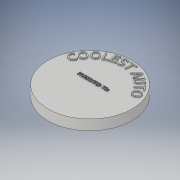
# Autodesk Inventor part: COOLEST AUTO
Saved by Autodesk Inventor 2018.2 (Build 222227000, 227)
## iProperties
Created: 2018-03-08
Part Number: COOLEST AUTO
Material: Generic
Document SubType Name: Modeling
Designer: battin.michael
Density: 1 g/cm^3
Appearance: Default
Author: battin.michael
Autodesk Inventor part; units mm, degrees
ref_plane "YZ Plane" through (0, 0, 0) normal (1, 0, 0) x (0, 1, 0)
ref_plane "XZ Plane" through (0, 0, 0) normal (0, 1, 0) x (-1, 0, 0)
ref_plane "XY Plane" through (0, 0, 0) normal (0, 0, 1) x (1, 0, 0)
sketch "Sketch1" plane through (0, 0, 0) normal (0, 1, 0) x (-1, 0, 0)
  circle A0 centre (0, 0) radius 104.775
  dimension "d0" = 209.55
  constraints: 1 centre point, 1 coincident
  measures "d0" diameter of A0
extrude "Extrusion1" add sketch "Sketch1" along normal blind 25.4
sketch "Sketch2" plane through (0, 25.4, 0) normal (0, 1, 0) x (1, 0, 0)
  circle A0 centre (0, 0) radius 104.775
  spline S0 degree 2 poles (-70.4833, 32.8422) (-71.2808, 31.0342) (-73.8501, 28.514) (-75.5622, 27.9374) knots 0 0 0 1 2 2 2
  spline S1 degree 2 poles (-75.5622, 27.9374) (-77.2593, 27.3541) (-81.4135, 27.7285) (-83.7638, 28.7652) knots 0 0 0 1 2 2 2
  spline S2 degree 2 poles (-83.7638, 28.7652) (-86.0991, 29.7952) (-89.0394, 32.5138) (-89.8217, 34.2086) knots 0 0 0 1 2 2 2
  spline S3 degree 2 poles (-89.8217, 34.2086) (-90.5804, 35.8751) (-90.5489, 39.4966) (-89.7182, 41.3799) knots 0 0 0 1 2 2 2
  spline S4 degree 2 poles (-89.7182, 41.3799) (-89.3062, 42.3141) (-88.3107, 43.8367) (-87.7941, 44.4367) knots 0 0 0 1 2 2 2
  spline S5 degree 2 poles (-87.7941, 44.4367) (-87.3324, 44.953) (-86.2234, 45.9576) (-85.6195, 46.4291) knots 0 0 0 1 2 2 2
  line L0 (-85.6195, 46.4291) -> (-82.6364, 45.1134)
  line L1 (-82.6364, 45.1134) -> (-82.7228, 44.9175)
  spline S6 degree 2 poles (-82.7228, 44.9175) (-83.1703, 44.719) (-84.4659, 44.0666) (-85.1983, 43.5078) knots 0 0 0 1 2 2 2
  spline S7 degree 2 poles (-85.1983, 43.5078) (-85.9023, 42.9724) (-87.1371, 41.5193) (-87.6156, 40.4346) knots 0 0 0 1 2 2 2
  spline S8 degree 2 poles (-87.6156, 40.4346) (-88.1406, 39.2443) (-88.0982, 36.688) (-87.5163, 35.4775) knots 0 0 0 1 2 2 2
  spline S9 degree 2 poles (-87.5163, 35.4775) (-86.9127, 34.2754) (-84.4204, 32.1323) (-82.6275, 31.3415) knots 0 0 0 1 2 2 2
  spline S10 degree 2 poles (-82.6275, 31.3415) (-80.7141, 30.4976) (-77.5516, 30.2006) (-76.2502, 30.5804) knots 0 0 0 1 2 2 2
  spline S11 degree 2 poles (-76.2502, 30.5804) (-74.9856, 30.9585) (-73.1278, 32.6408) (-72.6095, 33.8159) knots 0 0 0 1 2 2 2
  spline S12 degree 2 poles (-72.6095, 33.8159) (-72.1377, 34.8857) (-71.8609, 36.9413) (-71.9403, 37.8222) knots 0 0 0 1 2 2 2
  spline S13 degree 2 poles (-71.9403, 37.8222) (-72.033, 38.6729) (-72.4014, 40.0412) (-72.5614, 40.4537) knots 0 0 0 1 2 2 2
  line L2 (-72.5614, 40.4537) -> (-72.4816, 40.6345)
  line L3 (-72.4816, 40.6345) -> (-69.5286, 39.3321)
  spline S14 degree 2 poles (-69.5286, 39.3321) (-69.5148, 38.5881) (-69.4659, 37.2707) (-69.5638, 36.396) knots 0 0 0 1 2 2 2
  spline S15 degree 2 poles (-69.5638, 36.396) (-69.6514, 35.4628) (-69.9916, 33.9571) (-70.4833, 32.8422) knots 0 0 0 1 2 2 2
  spline S16 degree 2 poles (-72.6503, 63.2503) (-70.878, 63.3537) (-66.9523, 61.991) (-64.9309, 60.4597) knots 0 0 0 1 2 2 2
  spline S17 degree 2 poles (-64.9309, 60.4597) (-62.9621, 58.9681) (-60.5283, 55.5543) (-60.168, 53.7939) knots 0 0 0 1 2 2 2
  spline S18 degree 2 poles (-60.168, 53.7939) (-59.7949, 51.9412) (-60.7173, 48.4876) (-61.9205, 46.8994) knots 0 0 0 1 2 2 2
  spline S19 degree 2 poles (-61.9205, 46.8994) (-63.1634, 45.2587) (-66.2678, 43.4788) (-68.0831, 43.346) knots 0 0 0 1 2 2 2
  spline S20 degree 2 poles (-68.0831, 43.346) (-69.8654, 43.2294) (-73.7844, 44.6283) (-75.7794, 46.1397) knots 0 0 0 1 2 2 2
  spline S21 degree 2 poles (-75.7794, 46.1397) (-77.8139, 47.681) (-80.1458, 51.0384) (-80.5555, 52.8155) knots 0 0 0 1 2 2 2
  spline S22 degree 2 poles (-80.5555, 52.8155) (-80.9159, 54.5759) (-80.0329, 58.0593) (-78.7999, 59.6869) knots 0 0 0 1 2 2 2
  spline S23 degree 2 poles (-78.7999, 59.6869) (-77.547, 61.3407) (-74.3833, 63.117) (-72.6503, 63.2503) knots 0 0 0 1 2 2 2
  spline S24 degree 2 poles (-66.6313, 58.2152) (-68.2326, 59.4283) (-71.2403, 60.612) (-72.5314, 60.5985) knots 0 0 0 1 2 2 2
  spline S25 degree 2 poles (-72.5314, 60.5985) (-73.8587, 60.5917) (-76.0709, 59.4168) (-76.9261, 58.288) knots 0 0 0 1 2 2 2
  spline S26 degree 2 poles (-76.9261, 58.288) (-77.8111, 57.1199) (-78.3297, 54.7445) (-77.9706, 53.4189) knots 0 0 0 1 2 2 2
  spline S27 degree 2 poles (-77.9706, 53.4189) (-77.6309, 52.1493) (-75.6541, 49.5774) (-74.0791, 48.3842) knots 0 0 0 1 2 2 2
  spline S28 degree 2 poles (-74.0791, 48.3842) (-70.8896, 45.9679) (-65.4747, 46.0801) (-63.7743, 48.3245) knots 0 0 0 1 2 2 2
  spline S29 degree 2 poles (-63.7743, 48.3245) (-62.074, 50.569) (-63.4418, 55.7989) (-66.6313, 58.2152) knots 0 0 0 1 2 2 2
  spline S30 degree 2 poles (-54.5955, 79.3599) (-52.8533, 79.0184) (-49.391, 76.7204) (-47.8151, 74.7336) knots 0 0 0 1 2 2 2
  spline S31 degree 2 poles (-47.8151, 74.7336) (-46.2801, 72.7985) (-44.7739, 68.8858) (-44.8636, 67.0911) knots 0 0 0 1 2 2 2
  spline S32 degree 2 poles (-44.8636, 67.0911) (-44.964, 65.2039) (-46.718, 62.0892) (-48.279, 60.8509) knots 0 0 0 1 2 2 2
  spline S33 degree 2 poles (-48.279, 60.8509) (-49.8916, 59.5718) (-53.3416, 58.6217) (-55.1327, 58.9454) knots 0 0 0 1 2 2 2
  spline S34 degree 2 poles (-55.1327, 58.9454) (-56.8878, 59.2767) (-60.3345, 61.6081) (-61.89, 63.5691) knots 0 0 0 1 2 2 2
  spline S35 degree 2 poles (-61.89, 63.5691) (-63.4762, 65.5687) (-64.8979, 69.4013) (-64.8517, 71.2244) knots 0 0 0 1 2 2 2
  spline S36 degree 2 poles (-64.8517, 71.2244) (-64.762, 73.0191) (-63.0388, 76.1726) (-61.439, 77.4415) knots 0 0 0 1 2 2 2
  spline S37 degree 2 poles (-61.439, 77.4415) (-59.8135, 78.7309) (-56.307, 79.6628) (-54.5955, 79.3599) knots 0 0 0 1 2 2 2
  spline S38 degree 2 poles (-50.0212, 72.9837) (-51.2696, 74.5576) (-53.8875, 76.4535) (-55.1412, 76.7622) knots 0 0 0 1 2 2 2
  spline S39 degree 2 poles (-55.1412, 76.7622) (-56.4283, 77.0864) (-58.8635, 76.4999) (-59.973, 75.6198) knots 0 0 0 1 2 2 2
  spline S40 degree 2 poles (-59.973, 75.6198) (-61.1212, 74.709) (-62.2154, 72.5379) (-62.198, 71.1646) knots 0 0 0 1 2 2 2
  spline S41 degree 2 poles (-62.198, 71.1646) (-62.1854, 69.8504) (-60.9119, 66.8671) (-59.6839, 65.319) knots 0 0 0 1 2 2 2
  spline S42 degree 2 poles (-59.6839, 65.319) (-57.1973, 62.184) (-51.9253, 60.9432) (-49.7192, 62.6931) knots 0 0 0 1 2 2 2
  spline S43 degree 2 poles (-49.7192, 62.6931) (-47.5132, 64.443) (-47.5345, 69.8488) (-50.0212, 72.9837) knots 0 0 0 1 2 2 2
  line L4 (-28.2092, 73.1574) -> (-38.7803, 67.9735)
  line L5 (-38.7803, 67.9735) -> (-47.7271, 86.2179)
  line L6 (-47.7271, 86.2179) -> (-45.3024, 87.4069)
  line L7 (-45.3024, 87.4069) -> (-37.4142, 71.3211)
  line L8 (-37.4142, 71.3211) -> (-29.2678, 75.316)
  line L9 (-29.2678, 75.316) -> (-28.2092, 73.1574)
  line L10 (-26.1949, 73.808) -> (-31.5594, 93.4071)
  line L11 (-31.5594, 93.4071) -> (-19.2981, 96.7632)
  line L12 (-19.2981, 96.7632) -> (-18.6634, 94.4444)
  line L13 (-18.6634, 94.4444) -> (-28.32, 91.8012)
  line L14 (-28.32, 91.8012) -> (-26.8506, 86.4329)
  line L15 (-26.8506, 86.4329) -> (-17.8452, 88.8978)
  line L16 (-17.8452, 88.8978) -> (-17.2105, 86.579)
  line L17 (-17.2105, 86.579) -> (-26.2159, 84.1141)
  line L18 (-26.2159, 84.1141) -> (-24.2248, 76.8399)
  line L19 (-24.2248, 76.8399) -> (-14.5682, 79.483)
  line L20 (-14.5682, 79.483) -> (-13.9335, 77.1642)
  line L21 (-13.9335, 77.1642) -> (-26.1949, 73.808)
  spline S44 degree 2 poles (-5.3293, 77.5599) (-7.5308, 77.4102) (-10.6819, 78.1203) (-12.0902, 78.6848) knots 0 0 0 1 2 2 2
  line L22 (-12.0902, 78.6848) -> (-12.3202, 82.0692)
  line L23 (-12.3202, 82.0692) -> (-12.1231, 82.0826)
  spline S45 degree 2 poles (-12.1231, 82.0826) (-10.7075, 80.9244) (-7.2458, 79.7733) (-5.685, 79.8794) knots 0 0 0 1 2 2 2
  spline S46 degree 2 poles (-5.685, 79.8794) (-3.4507, 80.0312) (-1.2933, 82.0429) (-1.3971, 83.5708) knots 0 0 0 1 2 2 2
  spline S47 degree 2 poles (-1.3971, 83.5708) (-1.4797, 84.7865) (-2.7818, 86.2165) (-4.1053, 86.5061) knots 0 0 0 1 2 2 2
  spline S48 degree 2 poles (-4.1053, 86.5061) (-5.0597, 86.7053) (-6.645, 86.9607) (-7.8315, 87.1771) knots 0 0 0 1 2 2 2
  spline S49 degree 2 poles (-7.8315, 87.1771) (-8.9019, 87.385) (-10.6182, 88.1101) (-11.3047, 88.7401) knots 0 0 0 1 2 2 2
  spline S50 degree 2 poles (-11.3047, 88.7401) (-11.9748, 89.3712) (-12.7876, 91.1315) (-12.868, 92.3144) knots 0 0 0 1 2 2 2
  spline S51 degree 2 poles (-12.868, 92.3144) (-13.0355, 94.7787) (-9.4178, 98.3751) (-6.4442, 98.5772) knots 0 0 0 1 2 2 2
  spline S52 degree 2 poles (-6.4442, 98.5772) (-4.7356, 98.6933) (-1.6669, 98.2252) (-0.3255, 97.6727) knots 0 0 0 1 2 2 2
  line L24 (-0.3255, 97.6727) -> (-0.1066, 94.4526)
  line L25 (-0.1066, 94.4526) -> (-0.3038, 94.4392)
  spline S53 degree 2 poles (-0.3038, 94.4392) (-1.3334, 95.2605) (-4.4456, 96.3693) (-6.1049, 96.2566) knots 0 0 0 1 2 2 2
  spline S54 degree 2 poles (-6.1049, 96.2566) (-7.9778, 96.1293) (-10.1748, 94.2139) (-10.0777, 92.7846) knots 0 0 0 1 2 2 2
  spline S55 degree 2 poles (-10.0777, 92.7846) (-9.9906, 91.5032) (-8.5231, 90.068) (-7.2182, 89.8101) knots 0 0 0 1 2 2 2
  spline S56 degree 2 poles (-7.2182, 89.8101) (-6.3483, 89.6381) (-3.8273, 89.2153) (-2.9891, 89.0247) knots 0 0 0 1 2 2 2
  spline S57 degree 2 poles (-2.9891, 89.0247) (-0.8591, 88.5258) (1.2548, 86.0782) (1.3832, 84.1889) knots 0 0 0 1 2 2 2
  spline S58 degree 2 poles (1.3832, 84.1889) (1.4647, 82.9896) (0.6517, 80.6237) (-0.1643, 79.7595) knots 0 0 0 1 2 2 2
  spline S59 degree 2 poles (-0.1643, 79.7595) (-1.0733, 78.8064) (-3.4729, 77.6861) (-5.3293, 77.5599) knots 0 0 0 1 2 2 2
  line L26 (9.2058, 77.5726) -> (11.6281, 95.324)
  line L27 (11.6281, 95.324) -> (4.8735, 96.2457)
  line L28 (4.8735, 96.2457) -> (5.1985, 98.6278)
  line L29 (5.1985, 98.6278) -> (21.3836, 96.4192)
  line L30 (21.3836, 96.4192) -> (21.0585, 94.0371)
  line L31 (21.0585, 94.0371) -> (14.3039, 94.9588)
  line L32 (14.3039, 94.9588) -> (11.8816, 77.2075)
  line L33 (11.8816, 77.2075) -> (9.2058, 77.5726)
  line L34 (26.9284, 73.824) -> (42.0876, 88.9907)
  line L35 (42.0876, 88.9907) -> (45.0681, 87.5139)
  line L36 (45.0681, 87.5139) -> (42.1851, 66.265)
  line L37 (42.1851, 66.265) -> (39.6325, 67.5297)
  line L38 (39.6325, 67.5297) -> (40.5021, 73.439)
  line L39 (40.5021, 73.439) -> (33.5524, 76.8822)
  line L40 (33.5524, 76.8822) -> (29.3777, 72.6105)
  line L41 (29.3777, 72.6105) -> (26.9284, 73.824)
  line L42 (40.8615, 75.8337) -> (42.2907, 85.8027)
  line L43 (42.2907, 85.8027) -> (35.2399, 78.619)
  line L44 (35.2399, 78.619) -> (40.8615, 75.8337)
  spline S60 degree 2 poles (49.1597, 60.1417) (47.7701, 61.2778) (46.299, 63.6929) (46.1664, 65.0137) knots 0 0 0 1 2 2 2
  spline S61 degree 2 poles (46.1664, 65.0137) (46.0048, 66.507) (47.2052, 69.3541) (48.581, 71.0369) knots 0 0 0 1 2 2 2
  line L45 (48.581, 71.0369) -> (56.6066, 80.8532)
  line L46 (56.6066, 80.8532) -> (58.6973, 79.1438)
  line L47 (58.6973, 79.1438) -> (50.6718, 69.3276)
  spline S62 degree 2 poles (50.6718, 69.3276) (49.7754, 68.2312) (48.8468, 66.5231) (48.7522, 65.6008) knots 0 0 0 1 2 2 2
  spline S63 degree 2 poles (48.7522, 65.6008) (48.6517, 64.6195) (49.5735, 62.7811) (50.6189, 61.9265) knots 0 0 0 1 2 2 2
  spline S64 degree 2 poles (50.6189, 61.9265) (51.6005, 61.1239) (53.6618, 60.5233) (54.6037, 60.8168) knots 0 0 0 1 2 2 2
  spline S65 degree 2 poles (54.6037, 60.8168) (55.4887, 61.0929) (56.9678, 62.3296) (57.8329, 63.3878) knots 0 0 0 1 2 2 2
  line L48 (57.8329, 63.3878) -> (65.9001, 73.255)
  line L49 (65.9001, 73.255) -> (67.9909, 71.5457)
  line L50 (67.9909, 71.5457) -> (59.9653, 61.7294)
  spline S66 degree 2 poles (59.9653, 61.7294) (58.6208, 60.0849) (56.0401, 58.2812) (54.5421, 58.1659) knots 0 0 0 1 2 2 2
  spline S67 degree 2 poles (54.5421, 58.1659) (53.1854, 58.0414) (50.613, 58.9535) (49.1597, 60.1417) knots 0 0 0 1 2 2 2
  line L51 (60.6461, 49.2373) -> (74.7505, 60.2847)
  line L52 (74.7505, 60.2847) -> (70.5468, 65.6516)
  line L53 (70.5468, 65.6516) -> (72.4395, 67.1341)
  line L54 (72.4395, 67.1341) -> (82.512, 54.2742)
  line L55 (82.512, 54.2742) -> (80.6194, 52.7917)
  line L56 (80.6194, 52.7917) -> (76.4157, 58.1586)
  line L57 (76.4157, 58.1586) -> (62.3113, 47.1113)
  line L58 (62.3113, 47.1113) -> (60.6461, 49.2373)
  spline S68 degree 2 poles (89.9349, 34.5019) (89.195, 32.888) (86.1504, 30.0599) (83.85, 28.9928) knots 0 0 0 1 2 2 2
  spline S69 degree 2 poles (83.85, 28.9928) (81.6093, 27.9534) (77.4527, 27.4049) (75.7289, 27.9123) knots 0 0 0 1 2 2 2
  spline S70 degree 2 poles (75.7289, 27.9123) (73.9177, 28.4517) (71.3, 30.886) (70.4616, 32.6935) knots 0 0 0 1 2 2 2
  spline S71 degree 2 poles (70.4616, 32.6935) (69.5954, 34.5607) (69.4793, 38.1373) (70.2133, 39.8029) knots 0 0 0 1 2 2 2
  spline S72 degree 2 poles (70.2133, 39.8029) (70.9463, 41.4317) (74.0197, 44.2369) (76.2903, 45.2901) knots 0 0 0 1 2 2 2
  spline S73 degree 2 poles (76.2903, 45.2901) (78.6057, 46.3641) (82.6646, 46.8492) (84.4262, 46.3775) knots 0 0 0 1 2 2 2
  spline S74 degree 2 poles (84.4262, 46.3775) (86.1501, 45.8702) (88.8125, 43.4566) (89.6717, 41.6043) knots 0 0 0 1 2 2 2
  spline S75 degree 2 poles (89.6717, 41.6043) (90.5448, 39.7222) (90.63, 36.0949) (89.9349, 34.5019) knots 0 0 0 1 2 2 2
  spline S76 degree 2 poles (82.6651, 31.5472) (84.4875, 32.3925) (86.9435, 34.4939) (87.5371, 35.6405) knots 0 0 0 1 2 2 2
  spline S77 degree 2 poles (87.5371, 35.6405) (88.1536, 36.8159) (88.1534, 39.3208) (87.5575, 40.6055) knots 0 0 0 1 2 2 2
  spline S78 degree 2 poles (87.5575, 40.6055) (86.9408, 41.9349) (85.0861, 43.507) (83.7468, 43.8115) knots 0 0 0 1 2 2 2
  spline S79 degree 2 poles (83.7468, 43.8115) (82.4662, 44.107) (79.2677, 43.5672) (77.4752, 42.7357) knots 0 0 0 1 2 2 2
  spline S80 degree 2 poles (77.4752, 42.7357) (73.8452, 41.0519) (71.4048, 36.2169) (72.5897, 33.6625) knots 0 0 0 1 2 2 2
  spline S81 degree 2 poles (72.5897, 33.6625) (73.7746, 31.1081) (79.0352, 29.8634) (82.6651, 31.5472) knots 0 0 0 1 2 2 2
  constraints: 1 centre point, 1 coincident, 1 other
extrude "Extrusion2" add sketch "Sketch2" along normal blind 2.54 contours S0 S1 S2 S3 S4 S5 L0 L1 S6 S7 S8 S9 S10 S11 S12 S13 L2 L3 S14 S15 | S16 S17 S18 S19 S20 S21 S22 S23 | S30 S31 S32 S33 S34 S35 S36 S37 | L4 L5 L6 L7 L8 L9 | L10 L11 L12 L13 L14 L15 L16 L17 L18 L19 L20 L21 | S44 L22 L23 S45 S46 S47 S48 S49 S50 S51 S52 L24 L25 S53 S54 S55 S56 S57 S58 S59 | L26 L27 L28 L29 L30 L31 L32 L33 | L34 L35 L36 L37 L38 L39 L40 L41 | S60 S61 L45 L46 L47 S62 S63 S64 S65 L48 L49 L50 S66 S67 | L51 L52 L53 L54 L55 L56 L57 L58 | S68 S69 S70 S71 S72 S73 S74 S75
sketch "Sketch3" plane through (0, 25.4, 0) normal (0, 1, 0) x (1, 0, 0)
  circle A0 centre (0, 0) radius 104.775 projected
  line L0 (0, 0) -> (0, 5.5372)
  line L1 (104.775, 5.5372) -> (-104.775, 5.5372)
  spline S0 degree 2 poles (-32.6567, 10.8601) (-32.6567, 10.3661) (-33.0087, 9.4769) (-33.3236, 9.1681) knots 0 0 0 1 2 2 2
  spline S1 degree 2 poles (-33.3236, 9.1681) (-33.7188, 8.7791) (-34.7871, 8.3777) (-35.6022, 8.3777) knots 0 0 0 1 2 2 2
  line L2 (-35.6022, 8.3777) -> (-36.4605, 8.3777)
  line L3 (-36.4605, 8.3777) -> (-36.4605, 5.5372)
  line L4 (-36.4605, 5.5372) -> (-37.4732, 5.5372)
  line L5 (-37.4732, 5.5372) -> (-37.4732, 13.1572)
  line L6 (-37.4732, 13.1572) -> (-35.559, 13.1572)
  spline S2 degree 2 poles (-35.559, 13.1572) (-34.8797, 13.1572) (-33.9288, 12.9349) (-33.5644, 12.6817) knots 0 0 0 1 2 2 2
  spline S3 degree 2 poles (-33.5644, 12.6817) (-33.1384, 12.3915) (-32.6567, 11.4961) (-32.6567, 10.8601) knots 0 0 0 1 2 2 2
  spline S4 degree 2 poles (-33.7126, 10.8292) (-33.7126, 11.2244) (-33.9843, 11.8049) (-34.2622, 11.9901) knots 0 0 0 1 2 2 2
  spline S5 degree 2 poles (-34.2622, 11.9901) (-34.503, 12.1507) (-35.1452, 12.2803) (-35.6207, 12.2803) knots 0 0 0 1 2 2 2
  line L7 (-35.6207, 12.2803) -> (-36.4605, 12.2803)
  line L8 (-36.4605, 12.2803) -> (-36.4605, 9.2422)
  line L9 (-36.4605, 9.2422) -> (-35.7689, 9.2422)
  spline S6 degree 2 poles (-35.7689, 9.2422) (-35.1514, 9.2422) (-34.3919, 9.4398) (-34.1449, 9.6992) knots 0 0 0 1 2 2 2
  spline S7 degree 2 poles (-34.1449, 9.6992) (-33.9164, 9.9277) (-33.7126, 10.4649) (-33.7126, 10.8292) knots 0 0 0 1 2 2 2
  line L10 (-25.7962, 5.5372) -> (-27.1115, 5.5372)
  line L11 (-27.1115, 5.5372) -> (-29.5198, 8.5691)
  line L12 (-29.5198, 8.5691) -> (-30.6807, 8.5691)
  line L13 (-30.6807, 8.5691) -> (-30.6807, 5.5372)
  line L14 (-30.6807, 5.5372) -> (-31.6934, 5.5372)
  line L15 (-31.6934, 5.5372) -> (-31.6934, 13.1572)
  line L16 (-31.6934, 13.1572) -> (-29.7297, 13.1572)
  spline S8 degree 2 poles (-29.7297, 13.1572) (-29.0752, 13.1572) (-28.1921, 13.0152) (-27.7908, 12.7558) knots 0 0 0 1 2 2 2
  spline S9 degree 2 poles (-27.7908, 12.7558) (-27.3894, 12.4965) (-26.9263, 11.6875) (-26.9263, 11.0886) knots 0 0 0 1 2 2 2
  spline S10 degree 2 poles (-26.9263, 11.0886) (-26.9263, 10.2549) (-27.7784, 9.1249) (-28.5071, 8.8532) knots 0 0 0 1 2 2 2
  line L17 (-28.5071, 8.8532) -> (-25.7962, 5.5372)
  spline S11 degree 2 poles (-27.9822, 11.0083) (-27.9822, 11.3417) (-28.2168, 11.8543) (-28.4638, 12.021) knots 0 0 0 1 2 2 2
  spline S12 degree 2 poles (-28.4638, 12.021) (-28.68, 12.163) (-29.2543, 12.2803) (-29.6742, 12.2803) knots 0 0 0 1 2 2 2
  line L18 (-29.6742, 12.2803) -> (-30.6807, 12.2803)
  line L19 (-30.6807, 12.2803) -> (-30.6807, 9.4151)
  line L20 (-30.6807, 9.4151) -> (-29.7915, 9.4151)
  spline S13 degree 2 poles (-29.7915, 9.4151) (-29.3531, 9.4151) (-28.6553, 9.5695) (-28.4144, 9.8103) knots 0 0 0 1 2 2 2
  spline S14 degree 2 poles (-28.4144, 9.8103) (-28.1921, 10.0203) (-27.9822, 10.6131) (-27.9822, 11.0083) knots 0 0 0 1 2 2 2
  line L21 (-25.1911, 5.5372) -> (-25.1911, 13.1572)
  line L22 (-25.1911, 13.1572) -> (-20.4239, 13.1572)
  line L23 (-20.4239, 13.1572) -> (-20.4239, 12.2556)
  line L24 (-20.4239, 12.2556) -> (-24.1784, 12.2556)
  line L25 (-24.1784, 12.2556) -> (-24.1784, 10.1685)
  line L26 (-24.1784, 10.1685) -> (-20.6771, 10.1685)
  line L27 (-20.6771, 10.1685) -> (-20.6771, 9.2669)
  line L28 (-20.6771, 9.2669) -> (-24.1784, 9.2669)
  line L29 (-24.1784, 9.2669) -> (-24.1784, 6.4388)
  line L30 (-24.1784, 6.4388) -> (-20.4239, 6.4388)
  line L31 (-20.4239, 6.4388) -> (-20.4239, 5.5372)
  line L32 (-20.4239, 5.5372) -> (-25.1911, 5.5372)
  spline S15 degree 2 poles (-17.1882, 5.4013) (-18.0157, 5.4013) (-19.1766, 5.7472) (-19.6891, 5.9942) knots 0 0 0 1 2 2 2
  line L33 (-19.6891, 5.9942) -> (-19.6891, 7.2662)
  line L34 (-19.6891, 7.2662) -> (-19.615, 7.2662)
  spline S16 degree 2 poles (-19.615, 7.2662) (-19.1148, 6.7969) (-17.849, 6.2782) (-17.2623, 6.2782) knots 0 0 0 1 2 2 2
  spline S17 degree 2 poles (-17.2623, 6.2782) (-16.4225, 6.2782) (-15.5642, 6.976) (-15.5642, 7.5503) knots 0 0 0 1 2 2 2
  spline S18 degree 2 poles (-15.5642, 7.5503) (-15.5642, 8.0072) (-16.015, 8.5753) (-16.5028, 8.7173) knots 0 0 0 1 2 2 2
  spline S19 degree 2 poles (-16.5028, 8.7173) (-16.8548, 8.8161) (-17.4414, 8.952) (-17.8798, 9.0631) knots 0 0 0 1 2 2 2
  spline S20 degree 2 poles (-17.8798, 9.0631) (-18.275, 9.1681) (-18.8987, 9.4831) (-19.1395, 9.7362) knots 0 0 0 1 2 2 2
  spline S21 degree 2 poles (-19.1395, 9.7362) (-19.3742, 9.9894) (-19.6335, 10.6687) (-19.6335, 11.1133) knots 0 0 0 1 2 2 2
  spline S22 degree 2 poles (-19.6335, 11.1133) (-19.6335, 12.0395) (-18.1886, 13.2931) (-17.0709, 13.2931) knots 0 0 0 1 2 2 2
  spline S23 degree 2 poles (-17.0709, 13.2931) (-16.4287, 13.2931) (-15.2925, 13.0399) (-14.8047, 12.799) knots 0 0 0 1 2 2 2
  line L35 (-14.8047, 12.799) -> (-14.8047, 11.5887)
  line L36 (-14.8047, 11.5887) -> (-14.8788, 11.5887)
  spline S24 degree 2 poles (-14.8788, 11.5887) (-15.2431, 11.9222) (-16.3793, 12.4162) (-17.003, 12.4162) knots 0 0 0 1 2 2 2
  spline S25 degree 2 poles (-17.003, 12.4162) (-17.7069, 12.4162) (-18.5776, 11.7555) (-18.5776, 11.2182) knots 0 0 0 1 2 2 2
  spline S26 degree 2 poles (-18.5776, 11.2182) (-18.5776, 10.7366) (-18.0651, 10.1623) (-17.5834, 10.0326) knots 0 0 0 1 2 2 2
  spline S27 degree 2 poles (-17.5834, 10.0326) (-17.2623, 9.9462) (-16.3299, 9.7239) (-16.0211, 9.6313) knots 0 0 0 1 2 2 2
  spline S28 degree 2 poles (-16.0211, 9.6313) (-15.2369, 9.3904) (-14.5083, 8.4209) (-14.5083, 7.7108) knots 0 0 0 1 2 2 2
  spline S29 degree 2 poles (-14.5083, 7.7108) (-14.5083, 7.26) (-14.8726, 6.3955) (-15.1999, 6.093) knots 0 0 0 1 2 2 2
  spline S30 degree 2 poles (-15.1999, 6.093) (-15.5642, 5.7595) (-16.4904, 5.4013) (-17.1882, 5.4013) knots 0 0 0 1 2 2 2
  line L37 (-13.477, 5.5372) -> (-13.477, 13.1572)
  line L38 (-13.477, 13.1572) -> (-8.7099, 13.1572)
  line L39 (-8.7099, 13.1572) -> (-8.7099, 12.2556)
  line L40 (-8.7099, 12.2556) -> (-12.4643, 12.2556)
  line L41 (-12.4643, 12.2556) -> (-12.4643, 10.1685)
  line L42 (-12.4643, 10.1685) -> (-8.9631, 10.1685)
  line L43 (-8.9631, 10.1685) -> (-8.9631, 9.2669)
  line L44 (-8.9631, 9.2669) -> (-12.4643, 9.2669)
  line L45 (-12.4643, 9.2669) -> (-12.4643, 6.4388)
  line L46 (-12.4643, 6.4388) -> (-8.7099, 6.4388)
  line L47 (-8.7099, 6.4388) -> (-8.7099, 5.5372)
  line L48 (-8.7099, 5.5372) -> (-13.477, 5.5372)
  line L49 (-2.1458, 5.5372) -> (-3.282, 5.5372)
  line L50 (-3.282, 5.5372) -> (-6.6536, 12.1074)
  line L51 (-6.6536, 12.1074) -> (-6.6536, 5.5372)
  line L52 (-6.6536, 5.5372) -> (-7.5984, 5.5372)
  line L53 (-7.5984, 5.5372) -> (-7.5984, 13.1572)
  line L54 (-7.5984, 13.1572) -> (-6.1596, 13.1572)
  line L55 (-6.1596, 13.1572) -> (-3.0906, 7.1242)
  line L56 (-3.0906, 7.1242) -> (-3.0906, 13.1572)
  line L57 (-3.0906, 13.1572) -> (-2.1458, 13.1572)
  line L58 (-2.1458, 13.1572) -> (-2.1458, 5.5372)
  line L59 (1.1763, 5.5372) -> (1.1763, 12.2556)
  line L60 (1.1763, 12.2556) -> (-1.3801, 12.2556)
  line L61 (-1.3801, 12.2556) -> (-1.3801, 13.1572)
  line L62 (-1.3801, 13.1572) -> (4.7455, 13.1572)
  line L63 (4.7455, 13.1572) -> (4.7455, 12.2556)
  line L64 (4.7455, 12.2556) -> (2.1891, 12.2556)
  line L65 (2.1891, 12.2556) -> (2.1891, 5.5372)
  line L66 (2.1891, 5.5372) -> (1.1763, 5.5372)
  line L67 (5.5236, 5.5372) -> (5.5236, 13.1572)
  line L68 (5.5236, 13.1572) -> (10.2907, 13.1572)
  line L69 (10.2907, 13.1572) -> (10.2907, 12.2556)
  line L70 (10.2907, 12.2556) -> (6.5363, 12.2556)
  line L71 (6.5363, 12.2556) -> (6.5363, 10.1685)
  line L72 (6.5363, 10.1685) -> (10.0375, 10.1685)
  line L73 (10.0375, 10.1685) -> (10.0375, 9.2669)
  line L74 (10.0375, 9.2669) -> (6.5363, 9.2669)
  line L75 (6.5363, 9.2669) -> (6.5363, 6.4388)
  line L76 (6.5363, 6.4388) -> (10.2907, 6.4388)
  line L77 (10.2907, 6.4388) -> (10.2907, 5.5372)
  line L78 (10.2907, 5.5372) -> (5.5236, 5.5372)
  spline S31 degree 2 poles (17.4105, 9.341) (17.4105, 8.2974) (16.5645, 6.6178) (15.8544, 6.1485) knots 0 0 0 1 2 2 2
  spline S32 degree 2 poles (15.8544, 6.1485) (15.274, 5.7842) (14.0822, 5.5372) (13.1559, 5.5372) knots 0 0 0 1 2 2 2
  line L79 (13.1559, 5.5372) -> (11.4022, 5.5372)
  line L80 (11.4022, 5.5372) -> (11.4022, 13.1572)
  line L81 (11.4022, 13.1572) -> (13.1374, 13.1572)
  spline S33 degree 2 poles (13.1374, 13.1572) (14.2119, 13.1572) (15.4345, 12.8361) (15.8668, 12.552) knots 0 0 0 1 2 2 2
  spline S34 degree 2 poles (15.8668, 12.552) (16.6016, 12.0642) (17.4105, 10.4525) (17.4105, 9.341) knots 0 0 0 1 2 2 2
  spline S35 degree 2 poles (16.3546, 9.3534) (16.3546, 10.2302) (15.7741, 11.4714) (15.1999, 11.8234) knots 0 0 0 1 2 2 2
  spline S36 degree 2 poles (15.1999, 11.8234) (14.7923, 12.0642) (13.8722, 12.2803) (13.1868, 12.2803) knots 0 0 0 1 2 2 2
  line L82 (13.1868, 12.2803) -> (12.4149, 12.2803)
  line L83 (12.4149, 12.2803) -> (12.4149, 6.4141)
  line L84 (12.4149, 6.4141) -> (13.1868, 6.4141)
  spline S37 degree 2 poles (13.1868, 6.4141) (13.8599, 6.4141) (14.8788, 6.6302) (15.2925, 6.9204) knots 0 0 0 1 2 2 2
  spline S38 degree 2 poles (15.2925, 6.9204) (15.8235, 7.2786) (16.3546, 8.4642) (16.3546, 9.3534) knots 0 0 0 1 2 2 2
  line L85 (23.5609, 5.5372) -> (23.5609, 12.2556)
  line L86 (23.5609, 12.2556) -> (21.0044, 12.2556)
  line L87 (21.0044, 12.2556) -> (21.0044, 13.1572)
  line L88 (21.0044, 13.1572) -> (27.13, 13.1572)
  line L89 (27.13, 13.1572) -> (27.13, 12.2556)
  line L90 (27.13, 12.2556) -> (24.5736, 12.2556)
  line L91 (24.5736, 12.2556) -> (24.5736, 5.5372)
  line L92 (24.5736, 5.5372) -> (23.5609, 5.5372)
  spline S39 degree 2 poles (33.2989, 12.2865) (33.7312, 11.7802) (34.2128, 10.2982) (34.2128, 9.3472) knots 0 0 0 1 2 2 2
  spline S40 degree 2 poles (34.2128, 9.3472) (34.2128, 8.4209) (33.7435, 6.9204) (33.2989, 6.4141) knots 0 0 0 1 2 2 2
  spline S41 degree 2 poles (33.2989, 6.4141) (32.8296, 5.883) (31.5884, 5.3766) (30.8412, 5.3766) knots 0 0 0 1 2 2 2
  spline S42 degree 2 poles (30.8412, 5.3766) (30.0694, 5.3766) (28.8344, 5.9015) (28.3836, 6.4141) knots 0 0 0 1 2 2 2
  spline S43 degree 2 poles (28.3836, 6.4141) (27.9451, 6.9204) (27.4758, 8.4086) (27.4758, 9.3472) knots 0 0 0 1 2 2 2
  spline S44 degree 2 poles (27.4758, 9.3472) (27.4758, 10.3043) (27.9513, 11.7616) (28.3898, 12.2865) knots 0 0 0 1 2 2 2
  spline S45 degree 2 poles (28.3898, 12.2865) (28.8344, 12.7929) (30.0755, 13.3178) (30.8412, 13.3178) knots 0 0 0 1 2 2 2
  spline S46 degree 2 poles (30.8412, 13.3178) (31.6193, 13.3178) (32.8667, 12.7743) (33.2989, 12.2865) knots 0 0 0 1 2 2 2
  spline S47 degree 2 poles (33.1569, 9.3472) (33.1569, 10.1006) (32.8296, 11.2676) (32.5332, 11.6505) knots 0 0 0 1 2 2 2
  spline S48 degree 2 poles (32.5332, 11.6505) (32.2306, 12.0457) (31.3785, 12.4409) (30.8474, 12.4409) knots 0 0 0 1 2 2 2
  spline S49 degree 2 poles (30.8474, 12.4409) (30.2978, 12.4409) (29.4704, 12.058) (29.1555, 11.6505) knots 0 0 0 1 2 2 2
  spline S50 degree 2 poles (29.1555, 11.6505) (28.8529, 11.2615) (28.5318, 10.0882) (28.5318, 9.3472) knots 0 0 0 1 2 2 2
  spline S51 degree 2 poles (28.5318, 9.3472) (28.5318, 7.8467) (29.7915, 6.2535) (30.8474, 6.2535) knots 0 0 0 1 2 2 2
  spline S52 degree 2 poles (30.8474, 6.2535) (31.9033, 6.2535) (33.1569, 7.8467) (33.1569, 9.3472) knots 0 0 0 1 2 2 2
  line L93 (37.0163, 5.5372) -> (35.7936, 5.5372)
  line L94 (35.7936, 5.5372) -> (35.7936, 6.9945)
  line L95 (35.7936, 6.9945) -> (37.0163, 6.9945)
  line L96 (37.0163, 6.9945) -> (37.0163, 5.5372)
  line L97 (37.0163, 9.798) -> (35.7936, 9.798)
  line L98 (35.7936, 9.798) -> (35.7936, 11.2553)
  line L99 (35.7936, 11.2553) -> (37.0163, 11.2553)
  line L100 (37.0163, 11.2553) -> (37.0163, 9.798)
  dimension "d5" = 5.5372
  constraints: 4 end point, 1 horizontal, 1 vertical
  measures "d5" distance of L0.start L0.end
extrude "Extrusion3" add sketch "Sketch3" along normal blind 2.54 contours L1 L94 L95 L96 | L5 L6 S2 S3 S0 S1 L2 L3 L1 | S41 S42 L1 | L1 S42 S43 S44 S45 S46 S39 S40 S41 | L15 L16 S8 S9 S10 L17 L1 L11 L12 L13 | L1 L85 L86 L87 L88 L89 L90 L91 | L1 L80 L81 S33 S34 S31 S32 | L21 L22 L23 L24 L25 L26 L27 L28 L29 L30 L31 L1 | L1 L67 L68 L69 L70 L71 L72 L73 L74 L75 L76 L77 | S15 L33 L34 S16 S17 S18 S19 S20 S21 S22 S23 L35 L36 S24 S25 S26 S27 S28 S29 S30 L1 | L1 S30 S15 | L1 L59 L60 L61 L62 L63 L64 L65 | L37 L38 L39 L40 L41 L42 L43 L44 L45 L46 L47 L1 | L53 L54 L55 L56 L57 L58 L1 L50 L51 | L97 L98 L99 L100
body "Solid1"
